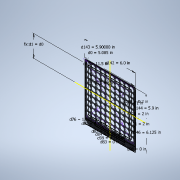
# Autodesk Inventor part: J009543
Saved by Autodesk Inventor 2020.3 (Build 243373000, 373)
## iProperties
RuleStatus: InUse
AfterDocSave0: file://Part Number Cleaner
Created: 2018-09-09
Material: DELRIN 100, BLACK (EXTRUDED)
Vendor: HHMI: JRC - ID&F
Document SubType Name: Modeling
Designer: arnoldj
Density: 1.42 g/cm^3
Appearance: Black Anodize
Part Number: J009543
Project: COMMON
Description: VP COMP LAYER H 10 x 10 V3
LAB/DEPT: COMMON
REQUESTING SCIENTIST: COMMON
SURFACE ROUGHNESS: 63 Ra
DESIGN DEPARTMENT: HHMI: JRC - ID&F
SPECIAL FINISH: NONE
ALTERED ITEM PART NUMBER: N/A
ALTERED ITEM VENDOR: N/A
ALTERED ITEM DESCRIPTION: N/A
Author: arnoldj
Revision Number: B
Autodesk Inventor part; units mm, degrees
ref_plane "YZ Plane" through (0, 0, 0) normal (1, 0, 0) x (0, 1, 0)
ref_plane "XZ Plane" through (0, 0, 0) normal (0, 1, 0) x (-1, 0, 0)
ref_plane "XY Plane" through (0, 0, 0) normal (0, 0, 1) x (1, 0, 0)
sketch "Sketch1" plane through (0, 0, 0) normal (0, 0, 1) x (1, 0, 0)
  line L0 (0, 210.947) -> (0, -216.662) projected
  line L1 (-210.312, 0) -> (212.852, 0) projected
  line L2 (152.4, -155.575) -> (-149.86, -155.575)
  line L3 (-149.86, -155.575) -> (-149.86, 149.86)
  line L4 (-149.86, 149.86) -> (152.4, 149.86)
  line L5 (152.4, 149.86) -> (152.4, -155.575)
  line L6 (129.159, -129.159) -> (-129.159, -129.159)
  line L7 (-129.159, -129.159) -> (-129.159, 129.159)
  line L8 (-129.159, 129.159) -> (129.159, 129.159)
  line L9 (129.159, 129.159) -> (129.159, -129.159)
  line L10 (129.159, -129.159) -> (-129.159, 129.159) construction
  line L11 (-129.159, -129.159) -> (129.159, 129.159) construction
  line L12 (76.2, -76.2) -> (-76.2, -76.2) construction
  line L13 (-76.2, -76.2) -> (-76.2, 76.2) construction
  line L14 (-76.2, 76.2) -> (76.2, 76.2) construction
  line L15 (76.2, 76.2) -> (76.2, -76.2) construction
  line L16 (76.2, -76.2) -> (-76.2, 76.2) construction
  line L17 (-76.2, -76.2) -> (76.2, 76.2) construction
  line L18 (114.808, -114.808) -> (-114.808, -114.808) construction
  line L19 (-114.808, -114.808) -> (-114.808, 114.808) construction
  line L20 (-114.808, 114.808) -> (114.808, 114.808) construction
  line L21 (114.808, 114.808) -> (114.808, -114.808) construction
  line L22 (114.808, -114.808) -> (-114.808, 114.808) construction
  line L23 (-114.808, -114.808) -> (114.808, 114.808) construction
  line L24 (146.05, -146.05) -> (-146.05, -146.05) construction
  line L25 (-146.05, -146.05) -> (-146.05, 146.05) construction
  line L26 (-146.05, 146.05) -> (146.05, 146.05) construction
  line L27 (146.05, 146.05) -> (146.05, -146.05) construction
  line L28 (146.05, -146.05) -> (-146.05, 146.05) construction
  line L29 (-146.05, -146.05) -> (146.05, 146.05) construction
  point P0 (0, 0)
  dimension "d0" = 129.159
  dimension "d1" = 129.159
  dimension "d23" = 152.4
  dimension "d36" = 114.808
  dimension "d63" = 292.1
  dimension "d142" = 152.4
  dimension "d143" = 149.86
  dimension "d144" = 149.86
  dimension "d146" = 155.575
  constraints: 56 end point, 10 parallel, 8 midpoint, 5 coincident, 5 horizontal, 5 perpendicular, 1 point on line
  measures "d0" distance from line of L0 L7.end
  measures "d1" distance from line of L1 L7.end
  measures "d23" distance of L13.end L14.end
  measures "d36" distance from line of L0 L19.end
  measures "d63" distance of L25.end L26.end
  measures "d142" distance between parallel lines of L0 L5
  measures "d143" distance between parallel lines of L0 L3
  measures "d144" distance between parallel lines of L1 L4
  measures "d146" distance between parallel lines of L1 L2
extrude "Extrusion1" add sketch "Sketch1" against normal blind 5.08
hole "Hole1" at (-129.159, 129.159, 0) direction (0, 0, -1) diameter 26.3398 end through all countersink diameter 28.575 countersink angle 60
chamfer "Chamfer5" [suppressed]
pattern_linear "Rectangular Pattern1" count 10 spacing 28.702 along (1, 0, 0) count 10 spacing 28.702 along (0, -1, 0) of "Hole1"
sketch "Sketch7" plane through (0, 0, -5.08) normal (0, 0, -1) x (-1, 0, 0)
  line L0 (0, -216.662) -> (0, 210.947) projected
  line L1 (-212.852, 0) -> (210.312, 0) projected
  point P0 (0, 0)
  point P1 (114.808, 114.808)
hole "Hole8-M4 CSINK" at (-114.808, 114.808, -5.08) direction (0, 0, 1) diameter 4.4958 end through all countersink diameter 9.525 countersink angle 90 clearance for "Flat Head Machine Screw" size "M4" standard "Ansi Metric M Profile"
pattern_linear "Rectangular Pattern3" count 5 spacing 57.404 along (1, 0, 0) count 5 spacing 57.404 along (0, -1, 0) of "Hole8-M4 CSINK"
sketch "Sketch4" plane through (0, 0, 0) normal (0, 0, 1) x (1, 0, 0)
  line L0 (152.4, -155.575) -> (-149.86, -155.575) projected
  line L1 (152.4, -184.15) -> (-149.86, -184.15)
  line L2 (-149.86, -184.15) -> (-149.86, -155.575)
  line L3 (-149.86, -155.575) -> (152.4, -155.575)
  line L4 (152.4, -155.575) -> (152.4, -184.15)
  line L5 (152.4, -184.15) -> (-149.86, -155.575) construction
  line L6 (-149.86, -184.15) -> (152.4, -155.575) construction
  line L7 (88.9, -165.1) -> (-88.9, -165.1)
  line L8 (-88.9, -165.1) -> (-88.9, -146.05)
  line L9 (-88.9, -146.05) -> (88.9, -146.05)
  line L10 (88.9, -146.05) -> (88.9, -165.1)
  line L11 (88.9, -165.1) -> (-88.9, -146.05) construction
  line L12 (-88.9, -165.1) -> (88.9, -146.05) construction
  line L13 (0, 216.662) -> (0, -250.952) projected
  line L14 (-210.312, 0) -> (212.852, 0) projected
  line L15 (152.4, 149.86) -> (152.4, -155.575) projected
  line L16 (152.4, 76.2) -> (147.32, 76.2)
  line L17 (147.32, 76.2) -> (147.32, 50.8)
  line L18 (147.32, 50.8) -> (152.4, 50.8)
  line L19 (152.4, 50.8) -> (152.4, 76.2)
  line L20 (152.4, -50.8) -> (147.32, -50.8)
  line L21 (147.32, -50.8) -> (147.32, -76.2)
  line L22 (147.32, -76.2) -> (152.4, -76.2)
  line L23 (152.4, -76.2) -> (152.4, -50.8)
  point P0 (0, 0)
  point P1 (1.27, -169.8625)
  point P2 (0, -155.575)
  point P3 (0, -178.5874)
  dimension "d76" = 28.575
  dimension "d82" = 177.8
  dimension "d83" = 0
  dimension "d84" = 19.05
  dimension "d85" = 19.05
  dimension "d98" = 0
  dimension "d99" = 5.5626
  dimension "d118" = 5.08
  dimension "d119" = 25.4
  dimension "d120" = 50.8
  dimension "d121" = 50.8
  constraints: 40 end point, 8 parallel, 4 horizontal, 4 midpoint, 4 perpendicular, 2 equal length, 2 point on line, 2 other
  measures "d76" distance of L1.end L0.end
  measures "d82" distance of L7.start L7.end
  measures "d84" distance between parallel lines of L7 L1
  measures "d85" distance of L7.end L8.end
  measures "d98" distance between parallel lines of L4 L15
  measures "d99" distance from line of L1 point (0, -178.587)
  measures "d118" distance of L16.start L16.end
  measures "d119" distance of L16.end L17.end
  measures "d120" distance between parallel lines of L18 L14
  measures "d121" distance between parallel lines of L20 L14
extrude "Extrusion4" add sketch "Sketch4" against normal up to surface (5.08 mm away) contours L4 L1 L13 L7 L10 L0 | L10 L7 L13 L0 | L13 L7 L8 L0 | L1 L2 L0 L8 L7 L13
sketch "Sketch5" plane through (0, 0, -5.08) normal (0, 0, -1) x (-1, 0, 0)
  point P0 (0, 0)
  point P1 (0, -178.5874)
  point P2 (101.6, -178.5874)
  dimension "d136" = 101.6
  constraints: 1 horizontal alignment
  measures "d136" distance of point (0, -178.587) point (101.6, -178.587)
hole "Hole6" at (0, -178.5874, -5.08) at (-101.6, -178.5874, -5.08) direction (0, 0, 1) diameter 3.81 end through all countersink diameter 7.0866 countersink angle 82 clearance for "Flat Head Machine Screw (82)" size "#6" standard "Ansi Unified Screw Threads"
chamfer "Chamfer9" distance 19.05 angle 15 1 edges at (-149.86, 149.86, -2.54) measured on face at (-149.86, -72.8133, -1.6933)
chamfer "Chamfer8" distance 19.05 angle 15 1 edges at (152.4, 149.86, -2.54) measured on face at (152.4, 38.5233, -3.3867)
fillet "Fillet7" radius 6.35 4 edges at (147.2956, 149.86, -2.54) (152.4, 130.81, -2.54) (-144.7556, 149.86, -2.54) (-149.86, 130.81, -2.54)
sketch "Sketch6" plane through (0, 0, 0) normal (0, 0, 1) x (1, 0, 0)
  line L0 (100.965, -173.99) -> (83.185, -173.99) construction
  line L1 (0, 199.6568) -> (0, -248.1178) construction
  line L2 (-30.48, 0) -> (182.88, 0) construction
  line L3 (152.4, 129.974) -> (152.4, -184.15) construction
  point P0 (0, 0)
  point P1 (92.075, -173.99)
  dimension "d126" = 17.78
  dimension "d127" = 173.99
  dimension "d147" = 92.075
  constraints: 2 coincident, 2 end point, 1 horizontal, 1 midpoint
  measures "d126" distance of L0.start L0.end
  measures "d127" distance between parallel lines of L0 L2
  measures "d147" distance from line of L1 point (92.075, -173.99)
hole "Hole7" at (100.965, -173.99, 0) at (83.185, -173.99, 0) direction (0, 0, -1) diameter 2.459 end through all thread size "M3x0.5" class "6H" standard "ANSI Metric M Profile"
fillet "Fillet8" radius 12.7 1 edges at (152.4, -184.15, -2.54)
chamfer "Chamfer10" distance 25.4 angle 45 1 edges at (-149.86, -184.15, -2.54)
fillet "Fillet9" radius 6.35 2 edges at (-149.86, -158.75, -2.54) (-124.46, -184.15, -2.54)
equation "\"d1\" = d0"
body "Solid1"
